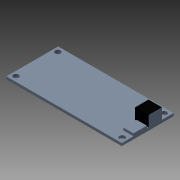
# Autodesk Inventor part: IOIO Board
Saved by Autodesk Inventor 2014 (Build 180170000, 170)
## iProperties
Created: 2013-09-05
Part Number: IOIO Board
Material: Allgemein
Document SubType Name: Modeling
Designer: vogel
Density: 1 g/cm^3
Appearance: Stahlblau
Author: vogel
Autodesk Inventor part; units mm, degrees
ref_plane "YZ Plane" through (0, 0, 0) normal (1, 0, 0) x (0, 1, 0)
ref_plane "XZ Plane" through (0, 0, 0) normal (0, 1, 0) x (-1, 0, 0)
ref_plane "XY Plane" through (0, 0, 0) normal (0, 0, 1) x (1, 0, 0)
sketch "Skizze1" plane through (0, 0, 0) normal (0, 0, 1) x (1, 0, 0)
  line L0 (-13.8, 0) -> (82.8, 0) projected
  line L1 (0, -6.2) -> (0, 37.2) projected
  line L2 (0, 0) -> (69, 0)
  line L3 (69, 0) -> (69, 31)
  line L4 (69, 31) -> (0, 31)
  line L5 (0, 31) -> (0, 0)
  line L6 (2.75, 28) -> (66.25, 28) construction
  line L7 (66.25, 28) -> (66.25, 3) construction
  line L8 (66.25, 3) -> (2.75, 3) construction
  line L9 (2.75, 3) -> (2.75, 28) construction
  circle A0 centre (2.75, 28) radius 1.65
  circle A1 centre (2.75, 3) radius 1.65
  circle A2 centre (66.25, 28) radius 1.65
  circle A3 centre (66.25, 3) radius 1.65
  dimension "d0" = 31
  dimension "d1" = 69
  dimension "d4" = 25
  dimension "d5" = 63.5
  dimension "d6" = 2.75
  dimension "d7" = 3
  dimension "d8" = 3.3
  constraints: 16 end point, 8 coincident, 4 centre point, 4 parallel, 3 equal radius, 2 horizontal, 2 perpendicular
  measures "d0" distance of L4.end L2.start
  measures "d1" distance of L2.start L2.end
  measures "d4" distance of L8.end L6.start
  measures "d5" distance of L6.start L6.end
  measures "d6" distance between parallel lines of L1 L9
  measures "d7" distance between parallel lines of L6 L4
  measures "d8" diameter of A0
extrude "Extrusion2" add sketch "Skizze1" along normal blind 1.6
sketch "Skizze2" plane through (0, 0, 1.6) normal (0, 0, 1) x (1, 0, 0)
  line L0 (69, 0) -> (69, 31) projected
  line L1 (69, 31) -> (0, 31) projected
  line L2 (69, 16) -> (61, 16)
  line L3 (61, 16) -> (61, 24)
  line L4 (61, 24) -> (69, 24)
  line L5 (69, 24) -> (69, 16)
  dimension "d11" = 15
  dimension "d12" = 8
  dimension "d13" = 8
  constraints: 8 end point, 2 parallel, 1 horizontal, 1 perpendicular, 1 point on line
  measures "d11" distance between parallel lines of L2 L1
  measures "d12" distance of L2.end L3.end
  measures "d13" distance of L3.end L4.end
extrude "Extrusion3" add sketch "Skizze2" along normal blind 6.5
sketch "Skizze3" plane through (0, 0, 1.6) normal (0, 0, 1) x (1, 0, 0)
  line L0 (0, 0) -> (69, 0) projected
  line L1 (69, 0) -> (69, 16) projected
  line L2 (69, 15) -> (63, 15)
  line L3 (63, 15) -> (63, 7)
  line L4 (63, 7) -> (69, 7)
  line L5 (69, 7) -> (69, 15)
  dimension "d16" = 8
  dimension "d17" = 6
  dimension "d18" = 15
  constraints: 8 end point, 2 parallel, 1 horizontal, 1 perpendicular, 1 point on line
  measures "d16" distance between parallel lines of L4 L2
  measures "d17" distance of L2.start L2.end
  measures "d18" distance between parallel lines of L0 L2
extrude "Extrusion4" add sketch "Skizze3" along normal blind 1.5
